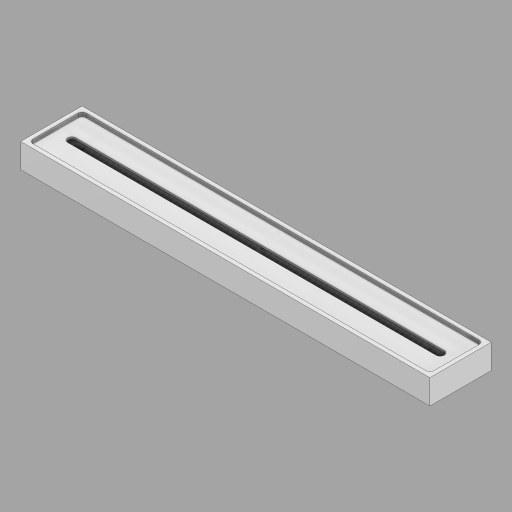
# Autodesk Inventor part: SolderSupport
Saved by Autodesk Inventor 2024 (Build 280153020, 153B)
## iProperties
Created: 2023-09-27
Part Number: SolderSupport
Material: Aluminum
Document SubType Name: Modeling
Designer: schanen
Density: 2.7 g/cm^3
Appearance: Satin
Author: schanen
Autodesk Inventor part; units mm, degrees
ref_plane "YZ Plane" through (0, 0, 0) normal (1, 0, 0) x (0, 1, 0)
ref_plane "XZ Plane" through (0, 0, 0) normal (0, 1, 0) x (-1, 0, 0)
ref_plane "XY Plane" through (0, 0, 0) normal (0, 0, 1) x (1, 0, 0)
sketch "Sketch1" plane through (0, 0, 0) normal (0, 1, 0) x (-1, 0, 0)
  line L0 (0, 0) -> (200, 0)
  line L1 (200, 0) -> (200, -30)
  line L2 (200, -30) -> (0, -30)
  line L3 (0, -30) -> (0, 0)
  line L4 (10, -15) -> (190, -15) construction
  line L5 (10, -13) -> (190, -13)
  line L6 (190, -17) -> (10, -17)
  arc A0 (10, -13) -> (10, -17) centre (10, -15) ccw
  arc A1 (190, -17) -> (190, -13) centre (190, -15) ccw
  point P0 (100, -15)
  dimension "d0" = 200
  dimension "d1" = 30
  dimension "d2" = 2
  dimension "d3" = 180
  dimension "d4" = 10
  dimension "d5" = 15
  constraints: 16 end point, 4 parallel, 4 point on circle, 4 tangent, 2 centre point, 1 horizontal, 1 midpoint, 1 perpendicular
  measures "d0" distance of L1.end L2.end
  measures "d1" distance of L0.end L1.end
  measures "d2" radius of A1
  measures "d3" distance of L6.start L6.end
  measures "d4" distance from line of L1 L4.end
  measures "d5" distance from line of L2 point (100, -15)
extrude "Extrusion1" add sketch "Sketch1" along normal blind 12
sketch "Sketch2" plane through (0, 0, 0) normal (0, -1, 0) x (1, 0, 0)
  arc A0 (-190, -13) -> (-190, -17) centre (-190, -15) ccw projected
  line L0 (-190, -15) -> (-10, -15) construction
  line L1 (-190, -17) -> (-10, -17) projected
  line L2 (-190, -21) -> (-10, -21)
  line L3 (-10, -9) -> (-190, -9)
  arc A1 (-190, -9) -> (-190, -21) centre (-190, -15) ccw
  arc A2 (-10, -21) -> (-10, -9) centre (-10, -15) ccw
  arc A3 (-10, -17) -> (-10, -13) centre (-10, -15) ccw projected
  point P0 (0, 0)
  point P1 (-100, -15)
  dimension "d10" = 12
  constraints: 8 end point, 4 point on circle, 4 tangent, 2 centre point, 2 coincident, 2 parallel, 1 midpoint
  measures "d10" diameter of A2
extrude "Extrusion2" cut sketch "Sketch2" against normal blind 9
sketch "Sketch3" plane through (0, 12, 0) normal (0, 1, 0) x (1, 0, 0)
  line L0 (-2, 2) -> (-198, 2)
  line L1 (-198, 2) -> (-198, 28)
  line L2 (-198, 28) -> (-2, 28)
  line L3 (-2, 28) -> (-2, 2)
  line L4 (-200, 0) -> (0, 0) projected
  line L5 (0, 0) -> (0, 30) projected
  line L6 (0, 30) -> (-200, 30) projected
  line L7 (-200, 30) -> (-200, 0) projected
  dimension "d13" = 2
  dimension "d14" = 2
  dimension "d15" = 2
  dimension "d16" = 2
  constraints: 8 end point, 2 parallel, 1 horizontal, 1 perpendicular
  measures "d13" distance between parallel lines of L4 L0
  measures "d14" distance between parallel lines of L5 L3
  measures "d15" distance between parallel lines of L6 L2
  measures "d16" distance between parallel lines of L7 L1
extrude "Extrusion3" cut sketch "Sketch3" against normal blind 2 contours L0 L1 L2 L3
fillet "Fillet1" radius 2 4 edges at (-198, 11, -28) (-198, 11, -2) (-2, 11, -28) (-2, 11, -2)
equation "\"d3\" = d0 - 2 * d4"
equation "\"d5\" = 0.5 * d1"
body "Solid1"
